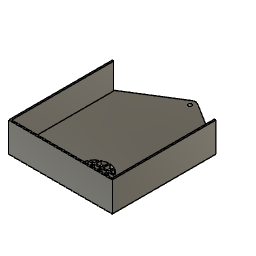
external cover v3 (Autodesk Fusion 360 design; units mm, degrees)
Autodesk Fusion 360 part; units mm, degrees
note: some values were not read from the file. Set by a fixed rule: which sketch regions a step uses.
sketch "Sketch1" plane through (0, 0, 0) normal (0, 0, 1) x (1, 0, 0)
  line L0 (70, 70) -> (-70, 70)
  line L1 (-70, 70) -> (-70, -70)
  line L2 (-70, -70) -> (70, -70)
  line L3 (70, -70) -> (70, 70)
  line L4 (70, 70) -> (-70, -70) construction
  line L5 (-70, 70) -> (70, -70) construction
  line L6 (0, 70) -> (0, 105)
  line L7 (0, 105) -> (0, 112.5)
  circle A0 centre (0, 105) radius 7.5
  line L8 (-70, 70) -> (-3.9815, 111.3559)
  line L9 (3.9815, 111.3559) -> (70, 70)
  circle A1 centre (0, 105) radius 2.5
  dimension "d1" = 140
  dimension "d2" = 140
  dimension "d3" = 35
  dimension "d4" = 7.5
  dimension "d5" = 5
  constraint horizontal L0
  constraint perpendicular L0 L1
  constraint parallel L0 L2
  constraint parallel L1 L3
  constraint coincident L4 origin
  constraint coincident L5 origin
  constraint midpoint L0 L6.start
  constraint perpendicular L0 L6
  constraint parallel L6 L7
  constraint coincident L6.end L7.start
  constraint coincident L7.end A0
  constraint coincident A0 L8.end
  constraint tangent A0 L8
  constraint coincident A0 L9.start
  constraint tangent A0 L9
  measures "d1" distance of L1.end L2.end
  measures "d2" distance of L0.start L2.end
  measures "d3" distance of L6.start L6.end
  measures "d4" distance of L6.end L7.end
  measures "d5" diameter of A1
extrude "Extrude1" add sketch "Sketch1" along normal blind 5 contours L0 L1 L2 L3 | L0 L6 A0 L9 | L0 L6 A0 L8 | L6 L7 A0 A1 | L6 L7 A0 A1
sketch "Sketch2" plane through (0, 0, 5) normal (0, 0, 1) x (-1, 0, 0)
  circle A0 centre (0, -105) radius 2.5
  line L0 (70, -70) -> (70, 70)
  line L1 (70, 70) -> (-70, 70)
  line L2 (-70, 70) -> (-70, -70)
  line L3 (-70, -70) -> (-3.9815, -111.3559)
  arc A1 (-3.9815, -111.3559) -> (3.9815, -111.3559) centre (0, -105) ccw
  line L4 (3.9815, -111.3559) -> (70, -70)
  line L5 (70, -70) -> (70, 70)
  line L6 (70, 70) -> (-70, 70)
  line L7 (-70, 70) -> (-70, -70)
  line L8 (68, 68) -> (-68, 68)
  line L9 (-68, 68) -> (-68, -68)
  line L10 (68, -68) -> (68, 68)
  line L11 (68, -68) -> (68, -70)
  line L12 (-68, -68) -> (-68, -70)
  line L13 (-70, -70) -> (-68, -70)
  line L14 (68, -70) -> (70, -70)
  dimension "d8" = 2
  dimension "d9" = 2
  dimension "d10" = 2
  constraint horizontal L13
  constraint vertical L5
  constraint horizontal L6
  constraint vertical L7
  constraint coincident L0.end L1.start
  constraint coincident L2.end L3.start
  constraint horizontal L8
  constraint vertical L9
  constraint vertical L10
  constraint coincident L11.end L13
  constraint perpendicular L11 L13
  constraint perpendicular L12 L13
  constraint collinear L13 L14
  measures "d8" distance of L7 L9
  measures "d9" distance of L6 L8
  measures "d10" distance of L5 L10
  measures "d18" diameter of A1.end
extrude "Extrude2" add sketch "Sketch2" along normal blind 35 contours L0 L1 L2 L5 L6 L7 L8 L9 L10 L11 L12 L13 L14
sketch "Sketch3" plane through (0, 0, 5) normal (0, 0, 1) x (-1, 0, 0)
  line L0 (-68, -70) -> (-70, -70)
  line L1 (-70, -70) -> (-3.9815, -111.3559)
  arc A0 (-3.9815, -111.3559) -> (3.9815, -111.3559) centre (0, -105) ccw
  line L2 (3.9815, -111.3559) -> (70, -70)
  line L3 (70, -70) -> (68, -70)
  line L4 (68, -70) -> (68, 68)
  line L5 (68, 68) -> (-68, 68)
  line L6 (-68, 68) -> (-68, -70)
  circle A1 centre (0, -105) radius 2.5
  circle A2 centre (-38, 38) radius 1.5
  line L7 (-38, 38) -> (10, 38)
  circle A3 centre (10, 38) radius 1.5
  circle A4 centre (-14, 38) radius 20
  line L8 (-14, 58) -> (-14, 18)
  line L9 (-13, 58) -> (-15, 58)
  line L10 (-15, 58) -> (-15, 18)
  line L11 (-15, 18) -> (-13, 18)
  line L12 (-13, 18) -> (-13, 58)
  line L13 (-13, 58) -> (-15, 18) construction
  line L14 (-15, 58) -> (-13, 18) construction
  line L15 (6, 37) -> (-34, 37)
  line L16 (-34, 37) -> (-34, 39)
  line L17 (-34, 39) -> (6, 39)
  line L18 (6, 39) -> (6, 37)
  line L19 (6, 37) -> (-34, 39) construction
  line L20 (-34, 37) -> (6, 39) construction
  line L21 (-14, 38) -> (-23.1711, 38)
  line L22 (-14, 38) -> (-23.1711, 38)
  line L23 (-24, 20.6795) -> (-24, 55.3205)
  line L24 (-24.1711, 55.2206) -> (-24.1711, 20.7794)
  line L25 (-22.1711, 19.7453) -> (-22.1711, 56.2547)
  line L26 (-22.9946, 55.8633) -> (-23.3458, 20.3179) construction
  line L27 (-23.3458, 55.6821) -> (-22.9946, 20.1367) construction
  line L28 (-14, 38) -> (-4, 38)
  line L29 (-5, 55.8606) -> (-5, 20.1394)
  line L30 (-3, 21.2967) -> (-3, 54.7033)
  line L31 (-3.3211, 54.9104) -> (-4.7111, 20.288) construction
  line L32 (-4.7111, 55.712) -> (-3.3211, 21.0896) construction
  line L33 (-14, 38) -> (-14, 48)
  line L34 (3.8606, 47) -> (-31.8606, 47)
  line L35 (-30.7033, 49) -> (2.7033, 49)
  line L36 (3.8606, 47) -> (-30.7443, 48.9375) construction
  line L37 (-31.8606, 47) -> (2.7443, 48.9375) construction
  line L38 (-14, 38) -> (-14, 28)
  line L39 (3.8606, 29) -> (-31.8606, 29)
  line L40 (-30.7033, 27) -> (2.7033, 27)
  line L41 (3.7436, 28.7715) -> (-30.8756, 27.2663) construction
  line L42 (-31.7436, 28.7715) -> (2.8756, 27.2663) construction
  point P0 (-14, 38)
  point P1 (-14, 38)
  point P2 (-23.1711, 38)
  point P3 (-4, 38)
  point P4 (-14, 48)
  point P5 (-14, 28)
  dimension "d14" = 3
  dimension "d15" = 30
  dimension "d16" = 30
  dimension "d17" = 48
  dimension "d18" = 3
  dimension "d19" = 40
  dimension "d22" = 40
  dimension "d23" = 2
  dimension "d24" = 40
  dimension "d25" = 2
  dimension "d27" = 10
  dimension "d30" = 10
  dimension "d32" = 10
  constraint coincident A2.centre L7.start
  constraint horizontal L7
  constraint coincident L7.end A3.centre
  constraint midpoint L7 P1
  constraint coincident A4 L8.start
  constraint coincident A4 L8.end
  constraint perpendicular L7 L8
  constraint horizontal L9
  constraint perpendicular L9 L10
  constraint parallel L9 L11
  constraint parallel L10 L12
  constraint coincident L13 P1
  constraint coincident L14 P1
  constraint coincident P1 P0
  constraint horizontal L15
  constraint perpendicular L15 L16
  constraint parallel L15 L17
  constraint parallel L16 L18
  constraint coincident L19 P1
  constraint coincident L20 P1
  constraint coincident L7 P2
  constraint parallel L7 L21
  constraint horizontal L22
  constraint coincident A4 L23.start
  constraint coincident A4 L23.end
  constraint perpendicular L15 L23
  constraint parallel L24 L25
  constraint coincident L26 P2
  constraint coincident L27 P2
  constraint coincident P2 L21.end
  constraint coincident A4 L25.end
  constraint coincident A4 L24.start
  constraint coincident A4 L26.start
  constraint coincident A4 L27.start
  constraint coincident A4 L25.start
  constraint coincident A4 L27.end
  constraint coincident A4 L24.end
  constraint coincident A4 L26.end
  constraint coincident L7 P3
  constraint parallel L7 L28
  constraint parallel L29 L30
  constraint coincident L31 P3
  constraint coincident L32 P3
  constraint coincident P3 L28.end
  constraint coincident A4 L30.end
  constraint coincident A4 L31.start
  constraint coincident A4 L32.start
  constraint coincident A4 L29.start
  constraint coincident A4 L30.start
  constraint coincident A4 L32.end
  constraint coincident A4 L31.end
  constraint coincident A4 L29.end
  constraint coincident L8 P4
  constraint perpendicular L22 L33
  constraint horizontal L34
  constraint parallel L34 L35
  constraint coincident L36 P4
  constraint coincident L37 P4
  constraint coincident A4 L34.start
  constraint coincident P4 L33.end
  constraint coincident A4 L37.end
  constraint coincident A4 L35.end
  constraint coincident A4 L36.end
  constraint coincident A4 L35.start
  constraint coincident L8 P5
  constraint horizontal L39
  constraint parallel L39 L40
  constraint coincident L41 P5
  constraint coincident L42 P5
  constraint coincident P5 L38.end
  constraint coincident A4 L40.end
  constraint coincident A4 L39.start
  constraint coincident A4 L42.end
  constraint coincident A4 L41.start
  constraint coincident A4 L40.start
  constraint coincident A4 L39.end
  constraint coincident A4 L42.start
  constraint coincident A4 L41.end
  measures "d14" diameter of A2
  measures "d15" distance of L6 A2.centre
  measures "d16" distance of L5 A2.centre
  measures "d17" distance of A2.centre L7.end
  measures "d18" diameter of A3
  measures "d19" diameter of A4
  measures "d22" distance of L9.start L11.end
  measures "d23" distance of L9.start L9.end
  measures "d24" distance of L15.start L15.end
  measures "d25" distance of L15.start L17.end
  measures "d27" distance of P1 P3
  measures "d30" distance of P1 P4
  measures "d32" distance of P1 P5
extrude "Extrude4" cut sketch "Sketch3" against normal blind 10 contours A2 | A4 L17 L24 L34 | A4 L15 L24 L39 | A4 L24 L35 | A4 L24 L40 | L10 L15 L25 L39 | L10 L17 L25 L34 | A4 L10 L25 L40 | A4 L10 L25 L35 | L12 L15 L29 L39 | L12 L17 L29 L34 | A4 L12 L29 L40 | A4 L15 L30 L39 | A4 L12 L29 L35 | A4 L17 L30 L34 | A4 L30 L40 | A4 L30 L35 | A3
extrude "Extrude3" [suppressed]
